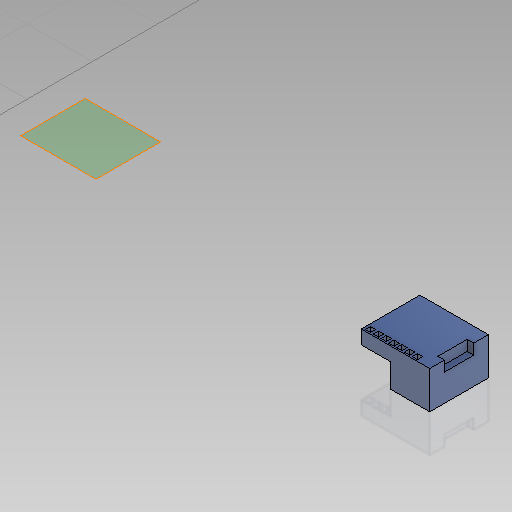
# Autodesk Inventor part: ЛЦМК0000002.00.00.00.00.04
Saved by Autodesk Inventor 2021.2 (Build 252289000, 289)
## iProperties
Created: 2025-10-23
Part Number: ЛЦМК0000002.00.00.00.00.04
Material: Типовые
Document SubType Name: Modeling
Designer: Захаров
Density: 1 g/cm^3
Appearance: С вкраплениями — сатинированная — синяя
Author: Захаров
Autodesk Inventor part; units mm, degrees
ref_plane "YZ Plane" through (0, 0, 0) normal (1, 0, 0) x (0, 1, 0)
ref_plane "XZ Plane" through (0, 0, 0) normal (0, 1, 0) x (-1, 0, 0)
ref_plane "XY Plane" through (0, 0, 0) normal (0, 0, 1) x (1, 0, 0)
ref_plane "РабПлоскость1" through (111.75, -2.8, -7.7) normal (0, -1, 0) x (1, 0, 0)
sketch "Эскиз1" plane through (111.75, -2.8, -7.7) normal (0, -1, 0) x (1, 0, 0)
  line L0 (99.15, 6.9) -> (97.55, 6.9) projected
  line L1 (97.55, 6.9) -> (97.55, 8.5) projected
  line L2 (97.55, 8.5) -> (99.15, 8.5) projected
  line L3 (99.15, 8.5) -> (99.15, 6.9) projected
  line L4 (94.35, 6.9) -> (92.75, 6.9) projected
  line L5 (92.75, 6.9) -> (92.75, 8.5) projected
  line L6 (92.75, 8.5) -> (94.35, 8.5) projected
  line L7 (94.35, 8.5) -> (94.35, 6.9) projected
  line L8 (103.95, 6.9) -> (102.35, 6.9) projected
  line L9 (102.35, 6.9) -> (102.35, 8.5) projected
  line L10 (102.35, 8.5) -> (103.95, 8.5) projected
  line L11 (103.95, 8.5) -> (103.95, 6.9) projected
  line L12 (101.55, 6.9) -> (99.95, 6.9) projected
  line L13 (99.95, 6.9) -> (99.95, 8.5) projected
  line L14 (99.95, 8.5) -> (101.55, 8.5) projected
  line L15 (101.55, 8.5) -> (101.55, 6.9) projected
  line L16 (106.35, 6.9) -> (104.75, 6.9) projected
  line L17 (104.75, 6.9) -> (104.75, 8.5) projected
  line L18 (104.75, 8.5) -> (106.35, 8.5) projected
  line L19 (106.35, 8.5) -> (106.35, 6.9) projected
  line L20 (96.75, 6.9) -> (95.15, 6.9) projected
  line L21 (95.15, 6.9) -> (95.15, 8.5) projected
  line L22 (95.15, 8.5) -> (96.75, 8.5) projected
  line L23 (96.75, 8.5) -> (96.75, 6.9) projected
  line L24 (108.75, 6.9) -> (107.15, 6.9) projected
  line L25 (107.15, 6.9) -> (107.15, 8.5) projected
  line L26 (107.15, 8.5) -> (108.75, 8.5) projected
  line L27 (108.75, 8.5) -> (108.75, 6.9) projected
  line L28 (111, 4.5) -> (113, 4.5) projected
  line L29 (113, 4.5) -> (113, 9) projected
  line L30 (113, 9) -> (92, 9) projected
  line L31 (92, 9) -> (92, -9) projected
  line L32 (92, -9) -> (113, -9) projected
  line L33 (113, -9) -> (113, -4.5) projected
  line L34 (113, -4.5) -> (111, -4.5) projected
  line L35 (111, -4.5) -> (111, 4.5) projected
  line L36 (97.55, -6.9) -> (99.15, -6.9) projected
  line L37 (99.15, -6.9) -> (99.15, -8.5) projected
  line L38 (99.15, -8.5) -> (97.55, -8.5) projected
  line L39 (97.55, -8.5) -> (97.55, -6.9) projected
  line L40 (92.75, -6.9) -> (94.35, -6.9) projected
  line L41 (94.35, -6.9) -> (94.35, -8.5) projected
  line L42 (94.35, -8.5) -> (92.75, -8.5) projected
  line L43 (92.75, -8.5) -> (92.75, -6.9) projected
  line L44 (102.35, -6.9) -> (103.95, -6.9) projected
  line L45 (103.95, -6.9) -> (103.95, -8.5) projected
  line L46 (103.95, -8.5) -> (102.35, -8.5) projected
  line L47 (102.35, -8.5) -> (102.35, -6.9) projected
  line L48 (99.95, -6.9) -> (101.55, -6.9) projected
  line L49 (101.55, -6.9) -> (101.55, -8.5) projected
  line L50 (101.55, -8.5) -> (99.95, -8.5) projected
  line L51 (99.95, -8.5) -> (99.95, -6.9) projected
  line L52 (104.75, -6.9) -> (106.35, -6.9) projected
  line L53 (106.35, -6.9) -> (106.35, -8.5) projected
  line L54 (106.35, -8.5) -> (104.75, -8.5) projected
  line L55 (104.75, -8.5) -> (104.75, -6.9) projected
  line L56 (95.15, -6.9) -> (96.75, -6.9) projected
  line L57 (96.75, -6.9) -> (96.75, -8.5) projected
  line L58 (96.75, -8.5) -> (95.15, -8.5) projected
  line L59 (95.15, -8.5) -> (95.15, -6.9) projected
  line L60 (107.15, -6.9) -> (108.75, -6.9) projected
  line L61 (108.75, -6.9) -> (108.75, -8.5) projected
  line L62 (108.75, -8.5) -> (107.15, -8.5) projected
  line L63 (107.15, -8.5) -> (107.15, -6.9) projected
  point P0 (-111.75, 7.7)
extrude "Выдавливание1" add sketch "Эскиз1" along normal blind 4.2 contours L35 L34 L33 L32 L31 L30 L29 L28 | L36 L37 L38 L39 | L40 L41 L42 L43 | L44 L45 L46 L47 | L48 L49 L50 L51 | L52 L53 L54 L55 | L56 L57 L58 L59 | L60 L61 L62 L63
sketch "Эскиз2" plane through (111.75, -7, -7.7) normal (0, -1, 0) x (1, 0, 0)
  line L0 (113, -9) -> (113, -4.5) projected
  line L1 (113, 9) -> (92, 9) projected
  line L2 (113, -9) -> (101, -9)
  line L3 (101, -9) -> (101, 9)
  line L4 (101, 9) -> (113, 9)
  line L5 (113, 9) -> (113, -9)
  point P0 (-111.75, 7.7)
  point P1 (113, 9)
  dimension "d2" = 12
  constraints: 8 end point, 2 parallel, 1 horizontal, 1 perpendicular, 1 point on line
  measures "d2" distance of L3.end L4.end
extrude "Выдавливание2" add sketch "Эскиз2" along normal blind 7.3
sketch "Эскиз3" plane through (111.75, -14.3, -7.7) normal (0, -1, 0) x (1, 0, 0)
  line L0 (97.55, 6.9) -> (99.15, 6.9) projected
  line L1 (99.15, 6.9) -> (99.15, 8.5) projected
  line L2 (99.15, 8.5) -> (97.55, 8.5) projected
  line L3 (97.55, 8.5) -> (97.55, 6.9) projected
  line L4 (92.75, 6.9) -> (94.35, 6.9) projected
  line L5 (94.35, 6.9) -> (94.35, 8.5) projected
  line L6 (94.35, 8.5) -> (92.75, 8.5) projected
  line L7 (92.75, 8.5) -> (92.75, 6.9) projected
  line L8 (102.35, 6.9) -> (103.95, 6.9) projected
  line L9 (103.95, 6.9) -> (103.95, 8.5) projected
  line L10 (103.95, 8.5) -> (102.35, 8.5) projected
  line L11 (102.35, 8.5) -> (102.35, 6.9) projected
  line L12 (99.95, 6.9) -> (101.55, 6.9) projected
  line L13 (101.55, 6.9) -> (101.55, 8.5) projected
  line L14 (101.55, 8.5) -> (99.95, 8.5) projected
  line L15 (99.95, 8.5) -> (99.95, 6.9) projected
  line L16 (104.75, 6.9) -> (106.35, 6.9) projected
  line L17 (106.35, 6.9) -> (106.35, 8.5) projected
  line L18 (106.35, 8.5) -> (104.75, 8.5) projected
  line L19 (104.75, 8.5) -> (104.75, 6.9) projected
  line L20 (95.15, 6.9) -> (96.75, 6.9) projected
  line L21 (96.75, 6.9) -> (96.75, 8.5) projected
  line L22 (96.75, 8.5) -> (95.15, 8.5) projected
  line L23 (95.15, 8.5) -> (95.15, 6.9) projected
  line L24 (107.15, 6.9) -> (108.75, 6.9) projected
  line L25 (108.75, 6.9) -> (108.75, 8.5) projected
  line L26 (108.75, 8.5) -> (107.15, 8.5) projected
  line L27 (107.15, 8.5) -> (107.15, 6.9) projected
  line L28 (113, 9) -> (92, 9) projected
  line L29 (113, -9) -> (113, 9) projected
  line L30 (92, -9) -> (113, -9) projected
  line L31 (92, 9) -> (92, -9) projected
  line L32 (99.15, -6.9) -> (97.55, -6.9) projected
  line L33 (97.55, -6.9) -> (97.55, -8.5) projected
  line L34 (97.55, -8.5) -> (99.15, -8.5) projected
  line L35 (99.15, -8.5) -> (99.15, -6.9) projected
  line L36 (94.35, -6.9) -> (92.75, -6.9) projected
  line L37 (92.75, -6.9) -> (92.75, -8.5) projected
  line L38 (92.75, -8.5) -> (94.35, -8.5) projected
  line L39 (94.35, -8.5) -> (94.35, -6.9) projected
  line L40 (103.95, -6.9) -> (102.35, -6.9) projected
  line L41 (102.35, -6.9) -> (102.35, -8.5) projected
  line L42 (102.35, -8.5) -> (103.95, -8.5) projected
  line L43 (103.95, -8.5) -> (103.95, -6.9) projected
  line L44 (101.55, -6.9) -> (99.95, -6.9) projected
  line L45 (99.95, -6.9) -> (99.95, -8.5) projected
  line L46 (99.95, -8.5) -> (101.55, -8.5) projected
  line L47 (101.55, -8.5) -> (101.55, -6.9) projected
  line L48 (106.35, -6.9) -> (104.75, -6.9) projected
  line L49 (104.75, -6.9) -> (104.75, -8.5) projected
  line L50 (104.75, -8.5) -> (106.35, -8.5) projected
  line L51 (106.35, -8.5) -> (106.35, -6.9) projected
  line L52 (96.75, -6.9) -> (95.15, -6.9) projected
  line L53 (95.15, -6.9) -> (95.15, -8.5) projected
  line L54 (95.15, -8.5) -> (96.75, -8.5) projected
  line L55 (96.75, -8.5) -> (96.75, -6.9) projected
  line L56 (108.75, -6.9) -> (107.15, -6.9) projected
  line L57 (107.15, -6.9) -> (107.15, -8.5) projected
  line L58 (107.15, -8.5) -> (108.75, -8.5) projected
  line L59 (108.75, -8.5) -> (108.75, -6.9) projected
  point P0 (-111.75, 7.7)
extrude "Выдавливание3" cut sketch "Эскиз3" against normal blind 7.3 contours L11 L10 L9 L8 | L15 L14 L13 L12 | L19 L18 L17 L16 | L27 L26 L25 L24
sketch "Эскиз4" plane through (111.75, -7, -7.7) normal (0, 1, 0) x (1, 0, 0)
  line L0 (111, -4.5) -> (113, -4.5) projected
  line L1 (113, 4.5) -> (113, -4.5) projected
  line L2 (113, 4.5) -> (111, 4.5) projected
  line L3 (111, 4.5) -> (111, -4.5) projected
  point P0 (-111.75, -7.7)
ref_plane "РабПлоскость2" through (10.25, -6, -12.2) normal (0, -1, 0) x (1, 0, 0)
extrude "Выдавливание4" add sketch "Эскиз4" along normal up to surface (1 mm away)
